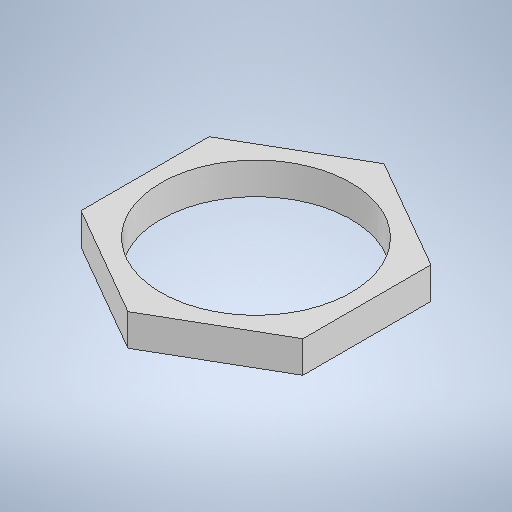
# Autodesk Inventor part: Nut
Saved by Autodesk Inventor 2025.2 (Build 292293000, 293)
## iProperties
Created: 2025-04-17
Part Number: Nut
Material: Generic
Document SubType Name: Modeling
Designer: Andreas
Density: 1 g/cm^3
Appearance: Default
Author: Andreas
Autodesk Inventor part; units mm, degrees
ref_plane "YZ Plane" through (0, 0, 0) normal (1, 0, 0) x (0, 1, 0)
ref_plane "XZ Plane" through (0, 0, 0) normal (0, 1, 0) x (-1, 0, 0)
ref_plane "XY Plane" through (0, 0, 0) normal (0, 0, 1) x (1, 0, 0)
sketch "Sketch1" plane through (0, 0, 0) normal (0, 1, 0) x (-1, 0, 0)
  line L0 (7, -4.0415) -> (0, -8.0829)
  line L1 (0, -8.0829) -> (-7, -4.0415)
  line L2 (-7, -4.0415) -> (-7, 4.0415)
  line L3 (-7, 4.0415) -> (0, 8.0829)
  line L4 (0, 8.0829) -> (7, 4.0415)
  line L5 (7, 4.0415) -> (7, -4.0415)
  circle A0 centre (0, 0) radius 6
  dimension "d0" = 14
  dimension "d1" = 12
  constraints: 12 end point, 2 coincident, 1 centre point, 1 vertical, 13 other
  measures "d0" distance between parallel lines of L2 L5
  measures "d1" diameter of A0
extrude "Extrusion1" add sketch "Sketch1" along normal blind 2
body "Solid1"
